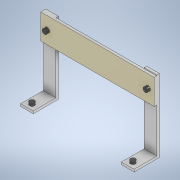
# Autodesk Inventor part: Frame
Saved by Autodesk Inventor 2021 (Build 250183000, 183)
## iProperties
Created: 2021-02-15
Part Number: Frame
Material: Generic
Document SubType Name: Modeling
Designer: Ryan
Density: 1 g/cm^3
Appearance: Default
Author: Ryan
Autodesk Inventor part; units mm, degrees
ref_plane "YZ Plane" through (0, 0, 0) normal (1, 0, 0) x (0, 1, 0)
ref_plane "XZ Plane" through (0, 0, 0) normal (0, 1, 0) x (-1, 0, 0)
ref_plane "XY Plane" through (0, 0, 0) normal (0, 0, 1) x (1, 0, 0)
sketch "Sketch1" plane through (0, 0, 0) normal (0, 1, 0) x (-1, 0, 0)
  line L0 (57.15, 25.4) -> (44.45, 25.4)
  line L1 (44.45, 25.4) -> (44.45, 0)
  line L2 (44.45, 0) -> (57.15, 0)
  line L3 (57.15, 0) -> (57.15, 25.4)
  line L4 (-44.45, 25.4) -> (-57.15, 25.4)
  line L5 (-57.15, 25.4) -> (-57.15, 0)
  line L6 (-57.15, 0) -> (-44.45, 0)
  line L7 (-44.45, 0) -> (-44.45, 25.4)
  line L8 (44.45, 25.4) -> (-44.45, 25.4) construction
  point P0 (0, 0)
  dimension "d0" = 12.7
  dimension "d1" = 25.4
  dimension "d2" = 114.3
  dimension "d3" = 57.15
  constraints: 18 end point, 4 parallel, 3 perpendicular, 3 point on line, 2 horizontal, 1 collinear
  measures "d0" distance of L0.start L0.end
  measures "d1" distance of L2.end L0.start
  measures "d2" distance between parallel lines of L5 L3
  measures "d3" distance from line of point (0, 0) L3
extrude "Extrusion1" add sketch "Sketch1" along normal blind 2.54
sketch "Sketch2" plane through (57.15, 0, 0) normal (0, 0, -1) x (-1, 0, 0)
  line L0 (0, 0.9525) -> (12.7, 0.9525)
  line L1 (12.7, 0.9525) -> (12.7, 73.3425)
  line L2 (12.7, 73.3425) -> (0, 73.3425)
  line L3 (0, 73.3425) -> (0, 0.9525)
  line L4 (101.6, 0) -> (114.3, 0)
  line L5 (114.3, 0) -> (114.3, 72.39)
  line L6 (114.3, 72.39) -> (101.6, 72.39)
  line L7 (101.6, 72.39) -> (101.6, 0)
  line L8 (12.7, 0) -> (12.7, 2.54) projected
  point P0 (57.15, 0)
  dimension "d6" = 12.7
  dimension "d7" = 12.7
  dimension "d8" = 12.7
  dimension "d9" = 72.39
  constraints: 16 end point, 5 parallel, 2 horizontal, 2 perpendicular
  measures "d6" distance of L0.start L0.end
  measures "d7" distance between parallel lines of L3 L8
  measures "d8" distance from line of L4.start L5
  measures "d9" distance of L0.end L1.end
extrude "Extrusion2" add sketch "Sketch2" against normal blind 2.54
sketch "Sketch3" plane through (57.15, 0, 2.54) normal (0, 0, 1) x (1, 0, 0)
  line L0 (-114.3, 72.39) -> (-114.3, 2.54) projected
  line L1 (0, 2.54) -> (0, 73.3425) projected
  line L2 (-114.3, 72.39) -> (0, 72.39)
  line L3 (0, 72.39) -> (0, 46.99)
  line L4 (0, 46.99) -> (-114.3, 46.99)
  line L5 (-114.3, 46.99) -> (-114.3, 72.39)
  point P0 (-57.15, 0)
  point P1 (0, 72.39)
  point P2 (0, 3.81)
  dimension "d12" = 25.4
  constraints: 8 end point, 2 parallel, 1 horizontal, 1 perpendicular, 1 point on line
  measures "d12" distance between parallel lines of L2 L4
extrude "Extrusion3" add sketch "Sketch3" along normal blind 2.54
sketch "Sketch4" plane through (57.15, 0, 5.08) normal (0, 0, 1) x (1, 0, 0)
  circle A0 centre (-107.95, 59.69) radius 2.54
  circle A1 centre (-6.35, 59.69) radius 2.54
  line L0 (-114.3, 72.39) -> (-114.3, 46.99) projected
  line L1 (-114.3, 59.69) -> (-107.95, 59.69)
  line L2 (-107.95, 59.69) -> (-6.35, 59.69)
  line L3 (-6.35, 59.69) -> (0, 59.69)
  line L4 (0, 46.99) -> (0, 72.39) projected
  point P0 (-57.15, 0)
  dimension "d15" = 5.08
  dimension "d16" = 6.35
  constraints: 6 end point, 2 centre point, 2 collinear, 2 midpoint, 1 equal radius, 1 perpendicular
  measures "d15" diameter of A0
  measures "d16" distance of L1.start L1.end
extrude "Extrusion4" add sketch "Sketch4" along normal blind 2.54
sketch "Sketch5" plane through (0, 2.54, 0) normal (0, 1, 0) x (1, 0, 0)
  circle A0 centre (-50.8, -20.32) radius 2.54
  circle A1 centre (50.8, -20.32) radius 2.54
  line L0 (-57.15, -25.4) -> (-44.45, -25.4) projected
  line L1 (-50.8, -25.4) -> (-50.8, 0) construction
  line L2 (44.45, -25.4) -> (57.15, -25.4) projected
  line L3 (50.8, -25.4) -> (50.8, 0) construction
  point P0 (0, 0)
  dimension "d19" = 5.08
  dimension "d20" = 5.08
  dimension "d21" = 5.08
  constraints: 4 end point, 2 centre point, 2 midpoint, 2 point on line, 2 vertical, 1 equal radius
  measures "d19" diameter of A0
  measures "d20" distance of L1.start A0.centre
  measures "d21" distance from line of L2 A1.centre
extrude "Extrusion5" add sketch "Sketch5" along normal blind 2.54
equation "\"d3\" = 0.5 * d2"
equation "\"d21\" = d20"
body "Solid1"
